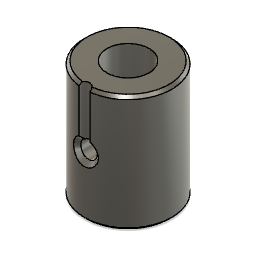
BearingWheelPin (Autodesk Fusion 360 design; units mm, degrees)
Autodesk Fusion 360 part; units mm, degrees
sketch "Sketch1" plane through (0, 0, 0) normal (0, 1, 0) x (1, 0, 0)
  circle A0 centre (0, 0) radius 3.95
  dimension "d1" = 7.9
  constraint coincident A0.centre origin
  measures "d1" diameter of A0
extrude "Extrude1" add sketch "Sketch1" along normal blind 10.5
chamfer "Chamfer1" distance 0.25 angle 45 2 edges at (-3.6827, 10.5, 1.4284) (-3.6827, 0, 1.4284)
hole "Hole1" at (0, 10.5, 0) direction (0, -1, 0) diameter 3.8 depth 20 tip angle 118
hole "Hole2" at (0, 5.3368, 3.95) direction (0, 0, -1) diameter 1.5 depth 3 tip angle 118
sketch "Sketch2" plane through (0, 10.5, 0) normal (0, 1, 0) x (-1, 0, 0)
  circle A0 centre (0, 0) radius 1.9
  circle A1 centre (0, 0) radius 3.7
  circle A2 centre (0, 0) radius 3.95
  circle A3 centre (0, 3.95) radius 0.5
  dimension "d11" = 1
  constraint coincident A2 A3.centre
  measures "d11" diameter of A3
extrude "Extrude2" cut sketch "Sketch2" against normal blind 4.5 contours A1 A3 | A1 A2 A3 | A2 A3 picked at (0, 3.6149) picked at (0.0466, 3.8634)
chamfer "Chamfer2" distance 0.3749 angle 45 2 edges at (0.7284, 5.1587, 3.8823) (-0.7284, 5.1587, 3.8823)
equation "d2 = 7.3 mm + 3.2 mm"
